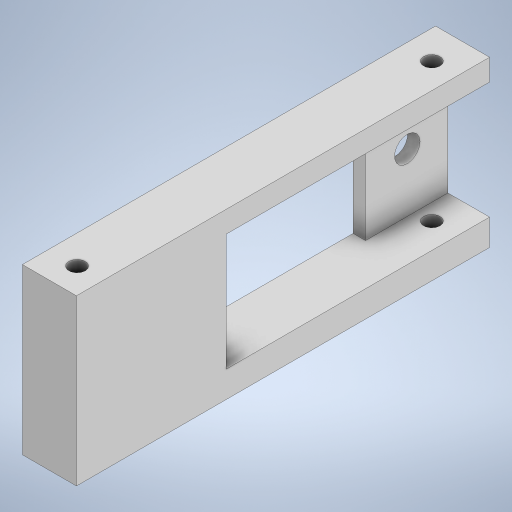
# Autodesk Inventor part: tcrt_to_mgn7
Saved by Autodesk Inventor 2024.2 (Build 282272000, 272)
## iProperties
Created: 2026-01-10
Part Number: tcrt_to_mgn7
Material: Типовые
Document SubType Name: Modeling
Designer: Service
Density: 1 g/cm^3
Appearance: По умолчанию
Author: Service
Autodesk Inventor part; units mm, degrees
ref_plane "YZ Plane" through (0, 0, 0) normal (1, 0, 0) x (0, 1, 0)
ref_plane "XZ Plane" through (0, 0, 0) normal (0, 1, 0) x (-1, 0, 0)
ref_plane "XY Plane" through (0, 0, 0) normal (0, 0, 1) x (1, 0, 0)
sketch "Эскиз1" plane through (0, 0, 0) normal (0, 1, 0) x (-1, 0, 0)
  circle A0 centre (0, 21.0368) radius 1
  circle A1 centre (0, -22.0362) radius 1
  line L0 (3.4815, 24.1933) -> (-3.0824, 24.1933)
  line L1 (-3.0824, 24.1933) -> (-3.0824, -25.9673)
  line L2 (-3.0824, -25.9673) -> (3.4815, -25.9673)
  line L3 (3.4815, -25.9673) -> (3.4815, 24.1933)
  point P0 (0, 0)
  dimension "d0" = 43.073
  dimension "d1" = 2
  dimension "d2" = 2
  constraints: 8 end point, 2 centre point, 2 parallel, 1 horizontal, 1 perpendicular
  measures "d0" distance of A0.centre A1.centre
  measures "d1" diameter of A0
  measures "d2" diameter of A1
extrude "Выдавливание1" add sketch "Эскиз1" along normal blind 20
sketch "Эскиз2" plane through (3.0824, 0, 24.1933) normal (1, 0, 0) x (0, 0, -1)
  line L0 (50.1606, 0) -> (50.1606, 20) projected
  line L1 (0, 0) -> (0, 20) projected
  line L2 (50.1606, 17.3924) -> (0, 17.3924)
  line L3 (0, 17.3924) -> (0, 3.1924)
  line L4 (0, 3.1924) -> (50.1606, 3.1924)
  line L5 (50.1606, 3.1924) -> (50.1606, 17.3924)
  line L6 (18.1606, 3.1924) -> (18.1606, 17.3924)
  line L7 (40.1606, 17.3924) -> (40.1606, 3.1924)
  line L8 (45.2295, 20) -> (45.2295, 0) projected
  circle A0 centre (45.2295, 10.2924) radius 1.55
  point P0 (24.1933, 0)
  point P1 (50.1606, 10)
  dimension "d5" = 14.2
  dimension "d6" = 32
  dimension "d7" = 10
  dimension "d8" = 3.1
  constraints: 12 end point, 7 point on line, 3 perpendicular, 2 parallel, 1 centre point, 1 horizontal, 1 midpoint
  measures "d5" distance between parallel lines of L4 L2
  measures "d6" distance between parallel lines of L6 L0
  measures "d7" distance from line of point (50.161, 10) L7
  measures "d8" diameter of A0
extrude "Выдавливание2" cut sketch "Эскиз2" against normal through all contours L4 L6 L2 L7 | A0 L8 | L8 A0
extrude "Выдавливание3" cut sketch "Эскиз2" against normal blind 5.064 contours L4 L8 A0 L2 L0 | L4 L7 L2 L8 A0
